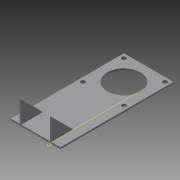
# Autodesk Inventor part: stepper_console_large
Saved by Autodesk Inventor 2015 SP1 (Build 190203100, 203)
## iProperties
Created: 2015-04-17
Part Number: stepper_console_large
Material: Ogólny
Document SubType Name: Modeling
Designer: Marcin
Density: 1 g/cm^3
Appearance: Domyślna
Author: Marcin
Autodesk Inventor part; units mm, degrees
ref_plane "YZ Plane" through (0, 0, 0) normal (1, 0, 0) x (0, 1, 0)
ref_plane "XZ Plane" through (0, 0, 0) normal (0, 1, 0) x (-1, 0, 0)
ref_plane "XY Plane" through (0, 0, 0) normal (0, 0, 1) x (1, 0, 0)
sketch "Szkic1" plane through (0, 0, 0) normal (0, 0, 1) x (1, 0, 0)
  line L0 (-28.5, -96.5) -> (28.5, -96.5)
  line L1 (28.5, -96.5) -> (28.5, 33.5)
  line L2 (28.5, 33.5) -> (-28.5, 33.5)
  line L3 (-28.5, 33.5) -> (-28.5, -96.5)
  line L4 (-28.5, -96.5) -> (28.5, 33.5) construction
  line L5 (28.5, -96.5) -> (-28.5, 33.5) construction
  line L6 (0, -96.5) -> (0, 33.5) construction
  line L7 (-26.5, 33.5) -> (26.5, 33.5) projected
  line L8 (26.5, -23.5) -> (-26.5, -23.5) projected
  line L9 (0, -23.5) -> (0, 33.5) construction
  point P0 (0, -31.5)
  dimension "d0" = 57
  dimension "d1" = 130
  constraints: 16 end point, 6 midpoint, 2 parallel, 1 horizontal, 1 perpendicular, 1 point on line
  measures "d0" distance of L0.start L0.end
  measures "d1" distance of L0.end L1.end
extrude "Wyciągnięcie proste1" add sketch "Szkic1" along normal blind 2
sketch "Szkic2" plane through (0, 0, 0) normal (0, 0, -1) x (-1, 0, 0)
  circle A0 centre (0, 5) radius 5 projected
  circle A1 centre (0, 5) radius 19.05 projected
  point P0 (0, 0)
extrude "Wyciągnięcie proste2" cut sketch "Szkic2" against normal blind 10 contours A0 | A1
sketch "Szkic3" plane through (0, 0, 0) normal (0, 0, -1) x (-1, 0, 0)
  circle A0 centre (-23.57, -18.57) radius 2.5 projected
  circle A1 centre (23.57, -18.57) radius 2.5 projected
  circle A2 centre (23.57, 28.57) radius 2.5 projected
  circle A3 centre (-23.57, 28.57) radius 2.5 projected
  point P0 (0, 0)
extrude "Wyciągnięcie proste3" cut sketch "Szkic3" against normal blind 10
ref_plane "Płaszczyzna konstrukcyjna1" through (18.5, -96.5, 0) normal (1, 0, 0) x (0, 0, -1)
sketch "Szkic5" plane through (18.5, -96.5, 0) normal (1, 0, 0) x (0, 0, -1)
  line L0 (-2, 0) -> (-27, 0)
  line L1 (-27, 0) -> (-2, 25)
  line L2 (-2, 0) -> (-2, 25)
  point P0 (0, 66.5)
  dimension "d14" = 25
  constraints: 6 end point, 1 horizontal, 1 perpendicular, 1 vertical
  measures "d14" distance of L0.start L1.end
extrude "Wyciągnięcie proste5" add sketch "Szkic5" against normal blind 2
mirror "Odbicie lustrzane1" about plane through (0, 0, 0) normal (1, 0, 0) of "Wyciągnięcie proste5"
